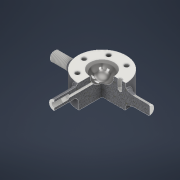
# Autodesk Inventor part: Test
Saved by Autodesk Inventor 2022 (Build 260153000, 153)
## iProperties
Created: 2023-05-24
Part Number: Test
Material: Чугун, литейный
Document SubType Name: Modeling
Designer: lxve_every1
Density: 7.15 g/cm^3
Appearance: Чугун — литейный
Author: lxve_every1
Autodesk Inventor part; units mm, degrees
ref_plane "XZ Plane" through (0, 0, 0) normal (0, 1, 0) x (-1, 0, 0)
ref_plane "XY Plane" through (0, 0, 0) normal (0, 0, 1) x (1, 0, 0)
sketch "Эскиз23" plane through (0, 0, 0) normal (0, 0, 1) x (1, 0, 0)
  circle A0 centre (0, 0) radius 50
  dimension "d150" = 100
  constraints: 1 centre point, 1 coincident
  measures "d150" diameter of A0
extrude "Выдавливание8" add sketch "Эскиз23" along normal blind 50
ref_plane "РабПлоскость16" through (0, 0, 25) normal (0, 0, 1) x (1, 0, 0)
sketch "Эскиз25" plane through (0, 0, 25) normal (0, 0, 1) x (1, 0, 0)
  line L0 (0, 0) -> (0, -100)
  line L1 (0, -100) -> (-10, -100)
  line L2 (-10, -100) -> (-10, -65)
  line L3 (-10, -65) -> (-15.3598, -44.997)
  line L4 (-15.3598, -44.997) -> (0, -44.997)
  dimension "d160" = 100
  dimension "d161" = 10
  dimension "d162" = 35
  dimension "d163" = 15
  constraints: 10 end point, 3 perpendicular, 1 point on line, 1 vertical
  measures "d160" distance of L0.start L0.end
  measures "d161" distance of L0.end L1.end
  measures "d162" distance of L1.end L2.end
  measures "d163" angle of L0 L3
revolve "Вращение8" add sketch "Эскиз25" angle 360 about axis through (0, 0, 25) along (0, 1, 0)
chamfer "Фаска8" distance 2 angle 45 1 edges at (14.6034, -47.8199, 24.9981)
thread "Резьба4" size "M20x2.5" class "6g" standard "ISO Metric profile" full length
chamfer "Фаска9" distance 2 angle 45 1 edges at (10, -100, 25)
mirror "Зеркальное отражение4" about plane through (0, 0, 0) normal (0, 1, 0) of "Вращение8", "Фаска8", "Фаска9"
sketch "Эскиз26" plane through (0, 0, 50) normal (0, 0, 1) x (1, 0, 0)
  circle A0 centre (0, 0) radius 25
  circle A1 centre (0, 0) radius 37.5
  line L0 (0, -25) -> (0, 25)
  dimension "d173" = 50
  dimension "d174" = 75
  constraints: 2 centre point, 2 coincident, 2 end point, 2 point on circle, 1 vertical
  measures "d173" diameter of A0
  measures "d174" diameter of A1
revolve "Вращение9" cut sketch "Эскиз26" angle 360 about axis through (0, -25, 50) along (0, -1, 0) picked at (-8.8525, -4.4917) contours L0 A0
ref_plane "РабПлоскость17" through (50, 0, 0) normal (1, 0, 0) x (0, 1, 0)
sketch "Эскиз29" plane through (50, 0, 0) normal (1, 0, 0) x (0, 1, 0)
  line L0 (0, 0) -> (0, 35)
  circle A0 centre (0, 35) radius 10
  dimension "d176" = 35
  dimension "d177" = 20
  constraints: 2 end point, 1 centre point, 1 coincident, 1 vertical
  measures "d176" distance of L0.start L0.end
  measures "d177" diameter of A0
extrude "Выдавливание9" add sketch "Эскиз29" along normal blind 50 and the other way blind 15.25
chamfer "Фаска10" distance 5 angle 45 3 edges at (48.9898, -10, 35.0018) (49.4151, 7.6255, 41.4693) (49.4151, 7.6255, 28.5307)
sketch "Эскиз30" plane through (100, 0, 35) normal (1, 0, 0) x (0, 0, -1)
  point P0 (35, 0)
  point P1 (0.0043, -0.0851)
hole "Отверстие6" at (100, -0.0851, 34.9957) direction (-1, 0, 0) diameter 10.106 depth 30 tip angle 120 countersink diameter 12 countersink angle 120 thread size "M12x1.75" class "6H" standard "ISO Metric profile"
sketch "Эскиз31" plane through (100, 0, 35) normal (1, 0, 0) x (0, 0, -1)
  circle A0 centre (0, 0) radius 2.5
  point P0 (35, 0)
  dimension "d192" = 5
  constraints: 1 centre point
  measures "d192" diameter of A0
extrude "Выдавливание10" cut sketch "Эскиз31" against normal blind 82.75
sketch "Эскиз32" plane through (0, 0, 50) normal (0, 0, 1) x (1, 0, 0)
  circle A0 centre (0, 0) radius 37.5
  line L0 (0, 0) -> (32.4314, -18.827)
  dimension "d195" = 75
  constraints: 2 end point, 1 coincident, 3 other
hole "Отверстие7" at (32.4314, -18.827, 50) direction (0, 0, -1) diameter 8.376 depth 20 tip angle 120 countersink diameter 10 countersink angle 120 thread size "M10x1.5" class "6H" standard "ISO Metric profile"
pattern_circular "Круговой массив4" count 6 over 360 about axis through (0, 0, 0) along (0, 0, 1) of "Отверстие7"
chamfer "Фаска11" distance 2 angle 45 1 edges at (-50, 0, 0)
